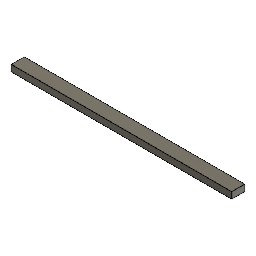
07part (Autodesk Fusion 360 design; units mm, degrees)
Autodesk Fusion 360 part; units mm, degrees
sketch "Sketch1" plane through (0, 0, 0) normal (1, 0, 0) x (0, 0, -1)
  line L0 (-18, 9) -> (18, 9)
  line L1 (18, 9) -> (18, -9)
  line L2 (18, -9) -> (-18, -9)
  line L3 (-18, -9) -> (-18, 9)
  dimension "d1" = 36
  dimension "d2" = 18
  constraint horizontal L0
  constraint vertical L1
  constraint horizontal L2
  constraint vertical L3
  constraint collinear origin L0.end L2.end
  constraint collinear origin L0.start L1.end
  measures "d1" distance of L0.start L0.end
  measures "d2" distance of L0.start L2.end
extrude "Extrude1" add sketch "Sketch1" along normal blind 600
